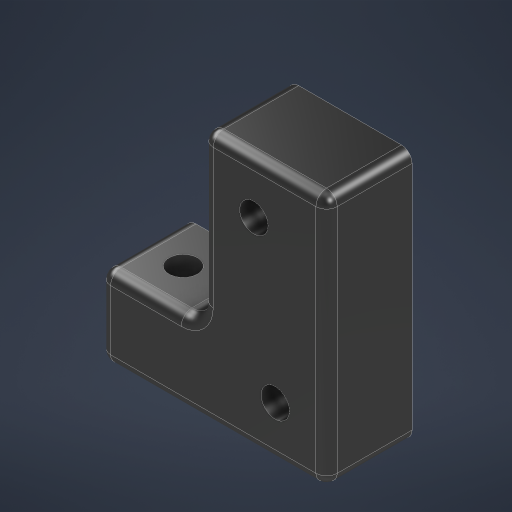
# Autodesk Inventor part: wing arm mount (left)
Saved by Autodesk Inventor 2024 (Build 280153000, 153)
## iProperties
Created: 2023-12-24
Part Number: wing arm mount (left)
Material: Generic
Document SubType Name: Modeling
Designer: elite
Density: 1 g/cm^3
Appearance: Glossy - Black
Author: elite
Autodesk Inventor part; units mm, degrees
ref_plane "YZ Plane" through (0, 0, 0) normal (1, 0, 0) x (0, 1, 0)
ref_plane "XZ Plane" through (0, 0, 0) normal (0, 1, 0) x (-1, 0, 0)
ref_plane "XY Plane" through (0, 0, 0) normal (0, 0, 1) x (1, 0, 0)
sketch "Sketch1" plane through (0, 0, 0) normal (0, 0, 1) x (1, 0, 0)
  line L0 (0, 0) -> (0, 22.225)
  line L1 (0, 22.225) -> (-3.175, 22.225)
  circle A0 centre (-3.175, 22.225) radius 2.1082
  circle A1 centre (0, 0) radius 2.1082
  line L2 (0, 0) -> (7.62, 0)
  line L3 (7.62, 0) -> (7.62, -7.62)
  line L4 (7.62, -7.62) -> (0, -7.62)
  line L5 (0, -7.62) -> (0, 0)
  line L6 (-3.175, 22.225) -> (-13.335, 22.225)
  line L7 (-13.335, 22.225) -> (-13.335, 29.845)
  line L8 (-13.335, 29.845) -> (-3.175, 29.845)
  line L9 (-3.175, 29.845) -> (-3.175, 22.225)
  line L10 (-13.335, 29.845) -> (7.62, 29.845)
  line L11 (7.62, 29.845) -> (7.62, -7.62)
  line L12 (7.62, -7.62) -> (-13.335, -7.62)
  line L13 (-13.335, -7.62) -> (-13.335, 29.845)
  line L14 (-13.335, 29.845) -> (-20.955, 29.845)
  line L15 (-20.955, 29.845) -> (-20.955, -7.62)
  line L16 (-20.955, -7.62) -> (-13.335, -7.62)
  line L17 (-13.335, -7.62) -> (-13.335, 29.845)
  point P0 (-3.175, 29.845)
  point P1 (-13.335, -7.62)
  dimension "d0" = 22.225
  dimension "d1" = 3.175
  dimension "d2" = 4.2164
  dimension "d3" = 4.2164
  dimension "d4" = 7.62
  dimension "d5" = 7.62
  dimension "d6" = 10.16
  dimension "d7" = 7.62
  dimension "d8" = 7.62
  constraints: 36 end point, 8 parallel, 5 perpendicular, 4 horizontal, 2 centre point, 2 coincident, 1 vertical
  measures "d0" distance of L0.start L0.end
  measures "d1" distance of L0.end L1.end
  measures "d2" diameter of A0
  measures "d3" diameter of A1
  measures "d4" distance of L3.end L4.end
  measures "d5" distance of L2.end L3.end
  measures "d6" distance of L7.end L8.end
  measures "d7" distance of L6.end L7.end
  measures "d8" distance of L15.end L16.end
extrude "Extrusion1" add sketch "Sketch1" along normal blind 12.7 contours A1 L5 L12 L13 L6 A0 L1 L0 | L0 L1 A0 L9 L10 L11 L2 A1 | L2 L3 L4 L5 A1 | L16 L15 L14 L7 L13 | A0 L6 L7 L8 L9
sketch "Sketch2" plane through (0, 0, 12.7) normal (0, 0, 1) x (1, 0, 0)
  line L0 (-20.955, 29.845) -> (-20.955, -7.62) projected
  line L1 (-20.955, 29.845) -> (-10.795, 29.845)
  line L2 (-10.795, 29.845) -> (-10.795, 4.445)
  line L3 (-10.795, 4.445) -> (-20.955, 4.445)
  line L4 (-20.955, 4.445) -> (-20.955, 29.845)
  point P0 (0, 0)
  point P1 (-20.955, 4.445)
  dimension "d11" = 10.16
  dimension "d12" = 25.4
  constraints: 8 end point, 2 parallel, 1 horizontal, 1 perpendicular
  measures "d11" distance of L2.end L3.end
  measures "d12" distance of L1.end L2.end
extrude "Extrusion2" cut sketch "Sketch2" against normal blind 31.75
fillet "Fillet1" radius 3.175 1 edges at (-10.795, 4.445, 6.35)
sketch "Sketch3" plane through (-20.955, -7.62, 0) normal (-1, 0, 0) x (0, 0, 1)
  point P0 (0, 7.62)
sketch "Sketch4" plane through (-20.955, -7.62, 0) normal (-1, 0, 0) x (0, 0, 1)
  line L0 (0, 12.065) -> (0, 0) projected
  line L1 (0, 12.065) -> (12.7, 12.065) projected
  line L2 (0, 0) -> (12.7, 0)
  line L3 (12.7, 0) -> (12.7, 12.065)
  line L4 (12.7, 12.065) -> (0, 12.065)
  line L5 (0, 12.065) -> (0, 0)
  point P0 (0, 7.62)
  constraints: 8 end point, 2 parallel, 1 horizontal, 1 perpendicular
extrude "Extrusion3" add sketch "Sketch4" along normal blind 5.08
sketch "Sketch5" plane through (-13.97, 4.445, 12.7) normal (0, 1, 0) x (1, 0, 0)
  line L0 (-12.065, 0) -> (-12.065, 12.7) projected
  line L1 (0, 0) -> (-12.065, 0) projected
  line L2 (-12.065, 12.7) -> (0, 0)
  circle A0 centre (-6.0325, 6.35) radius 2.1082
  point P0 (13.97, 12.7)
  dimension "d18" = 4.2164
  constraints: 2 end point, 1 centre point, 1 midpoint
  measures "d18" diameter of A0
extrude "Extrusion4" cut sketch "Sketch5" against normal blind 20.32 contours A0 L2 | L2 A0
fillet "Fillet2" radius 1.5875 12 edges at (-11.7249, 5.3749, 12.7) (-10.795, 18.7325, 12.7) (-20.0025, 4.445, 12.7) (-10.795, 29.845, 6.35) (-1.5875, 29.845, 12.7) (7.62, 29.845, 6.35) (7.62, 11.1125, 12.7) (-9.2075, -7.62, 12.7) (-26.035, -1.5875, 12.7) (-26.035, -7.62, 6.35) (-26.035, 4.445, 6.35) (7.62, -7.62, 6.35)
body "Solid1"
